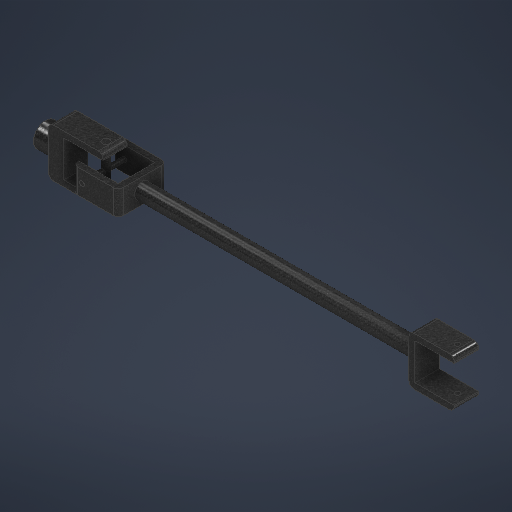
# Autodesk Inventor part: steeringcolumn
Saved by Autodesk Inventor 2026.2 (Build 302298010, 298A)
## iProperties
Created: 2026-07-06
Part Number: steeringcolumn
Material: Generic
Document SubType Name: Modeling
Designer: tasle
Density: 1 g/cm^3
Appearance: Default
Author: tasle
Autodesk Inventor part; units mm, degrees
ref_plane "YZ Plane" through (0, 0, 0) normal (1, 0, 0) x (0, 1, 0)
ref_plane "XZ Plane" through (0, 0, 0) normal (0, 1, 0) x (-1, 0, 0)
ref_plane "XY Plane" through (0, 0, 0) normal (0, 0, 1) x (1, 0, 0)
sketch "Sketch1" plane through (0, 0, 0) normal (0, 0, 1) x (1, 0, 0)
  line L0 (-195, 0) -> (195, 0)
  line L1 (-195, 0) -> (-170, 0)
  line L2 (-170, 0) -> (-170, 20)
  line L3 (-170, 20) -> (-195, 20)
  line L4 (-195, 20) -> (-195, 0)
  line L5 (-182.5, 25) -> (-170, 25)
  line L6 (-170, 25) -> (-170, -5)
  line L7 (-170, -5) -> (-182.5, -5)
  line L8 (-182.5, -5) -> (-182.5, 25)
  line L9 (-182.5, 25) -> (-137.5, 25)
  line L10 (-137.5, 25) -> (-137.5, 30)
  line L11 (-137.5, 30) -> (-182.5, 30)
  line L12 (-182.5, 30) -> (-182.5, 25)
  line L13 (-182.5, -5) -> (-137.5, -5)
  line L14 (-137.5, -5) -> (-137.5, -10)
  line L15 (-137.5, -10) -> (-182.5, -10)
  line L16 (-182.5, -10) -> (-182.5, -5)
  line L17 (-145, 30) -> (-145, -10)
  line L18 (-120, 20) -> (-115, 20)
  line L19 (-115, 20) -> (-115, 0)
  line L20 (-115, 0) -> (-120, 0)
  line L21 (-120, 0) -> (-120, 20)
  line L22 (0, 0) -> (0, 27.5)
  line L23 (120, 20) -> (115, 20)
  line L24 (115, 20) -> (115, 0)
  line L25 (115, 0) -> (120, 0)
  line L26 (120, 0) -> (120, 20)
  line L27 (-115, 16.5) -> (115, 16.5)
  line L28 (115, 16.5) -> (115, 3.5)
  line L29 (115, 3.5) -> (-115, 3.5)
  line L30 (-115, 3.5) -> (-115, 16.5)
  line L31 (-115, 10) -> (115, 10)
  line L32 (115, 30) -> (120, 30)
  line L33 (120, 30) -> (120, -10)
  line L34 (120, -10) -> (115, -10)
  line L35 (115, -10) -> (115, 30)
  point P0 (115, 0)
  dimension "d0" = 390
  dimension "d1" = 25
  dimension "d2" = 20
  dimension "d5" = 30
  dimension "d6" = 5
  dimension "d7" = 45
  dimension "d8" = 5
  dimension "d9" = 12.5
  dimension "d10" = 45
  dimension "d11" = 5
  dimension "d12" = 25
  dimension "d13" = 5
  dimension "d14" = 25
  dimension "d15" = 13
  dimension "d16" = 3.5
  dimension "d24" = 20
  dimension "d25" = 5
  dimension "d30" = 40
  dimension "d31" = 10
  constraints: 72 end point, 14 parallel, 8 horizontal, 8 perpendicular, 4 point on line, 4 symmetric about line, 3 midpoint, 1 vertical
  measures "d0" distance of L0.start L0.end
  measures "d1" distance of L3.end L2.end
  measures "d2" distance of L2.end L1.end
  measures "d5" distance of L5.end L6.end
  measures "d6" distance between parallel lines of L3 L5
  measures "d7" distance of L11.end L10.end
  measures "d8" distance of L10.end L9.end
  measures "d9" distance between parallel lines of L2 L8
  measures "d10" distance of L14.end L15.end
  measures "d11" distance of L13.end L14.end
  measures "d12" distance between parallel lines of L17 L2
  measures "d13" distance of L19.end L20.end
  measures "d14" distance between parallel lines of L21 L17
  measures "d15" distance between parallel lines of L29 L27
  measures "d16" distance between parallel lines of L18 L27
  measures "d24" distance of L20.end L18.start
  measures "d25" distance between parallel lines of L13 L20
  measures "d30" distance of L32.end L33.end
  measures "d31" distance between parallel lines of L23 L32
extrude "Extrusion1" add sketch "Sketch1" along normal mid plane 20 contours L8 L3 L2 L0 | L0 L6 L7 L8 | L7 L13 L17 L15 L16 | L8 L5 L6 L3 | L12 L11 L17 L9 L5 | L17 L11 L10 L9 | L13 L14 L15 L17
sketch "Sketch2" plane through (-182.5, -10, 10) normal (-1, 0, 0) x (0, 0, 1)
  circle A0 centre (-10, 20) radius 10
  point P0 (-10, 10)
  dimension "d19" = 20
  constraints: 1 centre point
  measures "d19" diameter of A0
extrude "Extrusion2" add sketch "Sketch2" along normal blind 12.5
extrude "Extrusion3" add sketch "Sketch1" along normal mid plane 40 separate body contours L21 L18 L19 L0
sketch "Sketch3" plane through (-120, 0, 20) normal (-1, 0, 0) x (0, 0, 1)
  line L0 (0, 0) -> (0, 20) projected
  line L1 (-40, 0) -> (0, 0) projected
  line L2 (0, 20) -> (-5, 20)
  line L3 (-5, 20) -> (-5, 0)
  line L4 (-5, 0) -> (0, 0)
  line L5 (0, 0) -> (0, 20)
  line L6 (-40, 20) -> (-35, 20)
  line L7 (-35, 20) -> (-35, 0)
  line L8 (-35, 0) -> (-40, 0)
  line L9 (-40, 0) -> (-40, 20)
  point P0 (-20, 0)
  dimension "d26" = 5
  dimension "d27" = 5
  constraints: 16 end point, 4 parallel, 3 point on line, 2 horizontal, 2 perpendicular
  measures "d26" distance of L4.end L3.end
  measures "d27" distance of L7.end L8.end
extrude "Extrusion4" add sketch "Sketch3" along normal blind 32.5 bodies 2
extrude "Extrusion5" add sketch "Sketch1" along normal mid plane 20 contours L24 L23 L26 L0 | L0 L33 L34 L35 | L23 L35 L32 L33 bodies 2
revolve "Revolution1" add sketch "Sketch1" angle 360 about axis through (-115, 10, 0) along (1, 0, 0) bodies 2 contours L19 L27 L22 L31 | L22 L27 L24 L31
sketch "Sketch4" plane through (120, -10, 10) normal (1, 0, 0) x (0, 0, -1)
  line L0 (20, 40) -> (0, 40) projected
  line L1 (20, 35) -> (20, 5) projected
  line L2 (0, 40) -> (20, 40)
  line L3 (20, 40) -> (20, 35)
  line L4 (20, 35) -> (0, 35)
  line L5 (0, 35) -> (0, 40)
  line L6 (20, 0) -> (0, 0) projected
  line L7 (0, 0) -> (20, 0)
  line L8 (20, 0) -> (20, 5)
  line L9 (20, 5) -> (0, 5)
  line L10 (0, 5) -> (0, 0)
  point P0 (10, 10)
  dimension "d35" = 5
  constraints: 16 end point, 4 parallel, 2 horizontal, 2 perpendicular, 1 point on line
  measures "d35" distance of L8.end L7.end
extrude "Extrusion6" add sketch "Sketch4" along normal blind 32.5 bodies 2
sketch "Sketch5" plane through (-195, 10, 0) normal (-1, 0, 0) x (0, 0, 1)
  arc A0 (-10, 0) -> (10, 0) centre (0, 0) ccw projected
  circle A1 centre (0, 0) radius 5
  point P0 (0, -10)
  dimension "d38" = 10
  constraints: 1 centre point, 1 coincident
  measures "d38" diameter of A1
extrude "Extrusion7" cut sketch "Sketch5" against normal blind 10 bodies 1
fillet "Fillet1" radius 4 12 edges at (-182.5, -10, 0) (-182.5, 30, 0) (-137.5, -10, 0) (-137.5, 30, 0) (-115, 10, 20) (-115, 10, -20) (115, 30, 0) (115, -10, 0) (152.5, 30, 0) (152.5, -10, 0) (-152.5, 10, 20) (-152.5, 10, -20)
sketch "Sketch6" plane through (-178.5, 30, -10) normal (0, 1, 0) x (1, 0, 0)
  circle A0 centre (33.5, -10) radius 3
  point P0 (178.5, -10)
  dimension "d42" = 6
  constraints: 1 centre point, 1 coincident
  measures "d42" diameter of A0
extrude "Extrusion8" cut sketch "Sketch6" against normal blind 51.275 bodies 1
sketch "Sketch7" plane through (0, 0, 20) normal (0, 0, 1) x (1, 0, 0)
  line L0 (-145, 30) -> (-145, -10) projected
  circle A0 centre (-145, 10) radius 2
  point P0 (0, 0)
  dimension "d45" = 4
  constraints: 1 centre point, 1 midpoint
  measures "d45" diameter of A0
extrude "Extrusion9" cut sketch "Sketch7" against normal blind 51.275 bodies 2
sketch "Sketch8" plane through (119, 30, -10) normal (0, 1, 0) x (1, 0, 0)
  circle A0 centre (26, -10) radius 2
  line L0 (29.5, 0) -> (29.5, -20) projected
  point P0 (-119, -10)
  dimension "d48" = 4
  dimension "d49" = 3.5
  constraints: 1 centre point
  measures "d48" diameter of A0
  measures "d49" distance from line of L0 A0.centre
extrude "Extrusion10" cut sketch "Sketch8" against normal blind 51.275 bodies 2
extrude "Extrusion11" add sketch "Sketch6" against normal up to surface (40 mm away) separate body
extrude "Extrusion12" cut sketch "Sketch7" against normal blind 35.4 bodies 3
extrude "Extrusion13" add sketch "Sketch7" against normal up to surface (40 mm away) separate body
